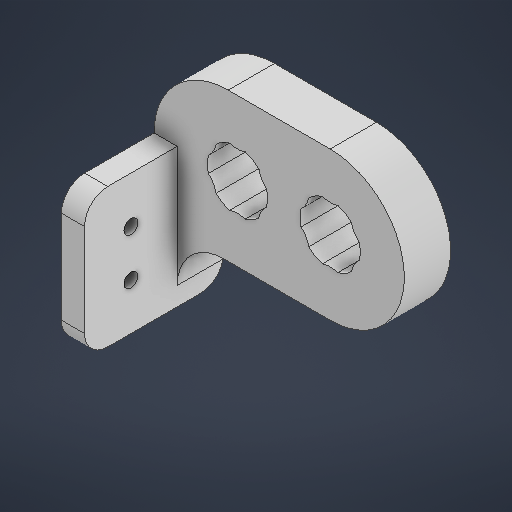
# Autodesk Inventor part: left_holder
Saved by Autodesk Inventor 2026.1 (Build 301233020, 233B)
## iProperties
Created: 2025-12-21
Part Number: left_holder
Material: Ogólny
Document SubType Name: Modeling
Designer: maciej
Density: 1 g/cm^3
Appearance: Domyślna
Author: maciej
Autodesk Inventor part; units mm, degrees
ref_plane "YZ Plane" through (0, 0, 0) normal (1, 0, 0) x (0, 1, 0)
ref_plane "XZ Plane" through (0, 0, 0) normal (0, 1, 0) x (-1, 0, 0)
ref_plane "XY Plane" through (0, 0, 0) normal (0, 0, 1) x (1, 0, 0)
sketch "Sketch1" plane through (0, 0, 0) normal (0, 0, 1) x (1, 0, 0)
  circle A0 centre (0, 0) radius 9.25
  circle A1 centre (0, 30) radius 6
  circle A2 centre (20, 30) radius 6
  circle A3 centre (0, 30) radius 6.5
  circle A4 centre (20, 30) radius 6.5
  arc A5 (-1.6614, 36.2841) -> (1.6614, 36.2841) centre (0, 41) ccw
  arc A6 (-6.2729, 31.7032) -> (-4.6115, 34.5808) centre (-9.5263, 35.5) ccw
  arc A7 (-4.6115, 25.4192) -> (-6.2729, 28.2968) centre (-9.5263, 24.5) ccw
  arc A8 (1.6614, 23.7159) -> (-1.6614, 23.7159) centre (0, 19) ccw
  arc A9 (6.2729, 28.2968) -> (4.6115, 25.4192) centre (9.5263, 24.5) ccw
  arc A10 (4.6115, 34.5808) -> (6.2729, 31.7032) centre (9.5263, 35.5) ccw
  arc A11 (18.3386, 36.2841) -> (21.6614, 36.2841) centre (20, 41) ccw
  arc A12 (13.7271, 31.7032) -> (15.3885, 34.5808) centre (10.4737, 35.5) ccw
  arc A13 (15.3885, 25.4192) -> (13.7271, 28.2968) centre (10.4737, 24.5) ccw
  arc A14 (21.6614, 23.7159) -> (18.3386, 23.7159) centre (20, 19) ccw
  arc A15 (26.2729, 28.2968) -> (24.6115, 25.4192) centre (29.5263, 24.5) ccw
  arc A16 (24.6115, 34.5808) -> (26.2729, 31.7032) centre (29.5263, 35.5) ccw
  arc A17 (4.6562, 34.5353) -> (4.5, 33.9686) centre (20, 30) ccw
  arc A18 (20, 14) -> (20, 46) centre (20, 30) ccw
  line L0 (-18, 30) -> (-18, 0)
  line L1 (-2, 46) -> (20, 46)
  line L2 (-18, 0) -> (-13, 0)
  line L3 (-13, 0) -> (-13, 30)
  line L4 (-13, 30) -> (-18, 30)
  line L5 (-18, 30) -> (-18, 0)
  arc A19 (-2, 46) -> (-18, 30) centre (-2, 30) ccw
  line L6 (20, 14) -> (-13, 14)
  point P0 (15.2791, 25.532)
  point P1 (-18, 30)
  point P2 (-1.6614, 23.7159)
  point P3 (1.6614, 23.7159)
  point P4 (-6.2729, 28.2968)
  point P5 (-4.6115, 25.4192)
  point P6 (-4.6115, 34.5808)
  point P7 (4.635, 34.4629)
  point P8 (6.2729, 31.7032)
  point P9 (18.3386, 23.7159)
  point P10 (21.6614, 23.7159)
  point P11 (13.7271, 31.7032)
  point P12 (26.2729, 31.7032)
  point P13 (15.3885, 25.4192)
  point P14 (15.3885, 34.5808)
  point P15 (4.6115, 25.4192)
  dimension "d1" = 12
  dimension "d0" = 18.5
  dimension "d2" = 30
  dimension "d3" = 12
  dimension "d4" = 20
  dimension "d5" = 13
  dimension "d6" = 13
  dimension "d7" = 5
  dimension "d10" = 360
  dimension "d12" = 5
  dimension "d15" = 360
  dimension "d21" = 16
  dimension "d25" = 5
  dimension "d26" = 30
  dimension "d52" = 18
  constraints: 36 point on circle, 19 centre point, 14 end point, 5 tangent, 4 coincident, 3 horizontal, 3 vertical alignment, 2 horizontal alignment, 2 parallel, 1 perpendicular, 1 point on line, 1 vertical, 54 other
  measures "d0" diameter of A0
  measures "d2" distance of point (0, 0) point (0, 30)
  measures "d3" diameter of A2
  measures "d4" distance of A2.centre point (0, 30)
  measures "d5" diameter of A3
  measures "d6" diameter of A4
  measures "d7" radius of A5
  measures "d12" radius of A11
  measures "d21" radius of A18
  measures "d25" distance of L0.start L3.end
  measures "d26" distance of L3.end L2.end
  measures "d52" distance from line of L0 point (0, 0)
extrude "Extrusion1" add sketch "Sketch1" along normal blind 10 contours A10 A17 A3 | A9 A3 | A8 A3 | A5 A3 | A7 A3 | A6 A3 | A16 A4 | A15 A4 | A11 A4 | A14 A4 | A12 A4 | A13 A4 | L6 L3 L4 A19 L1 A18 | L3 L2 L0 L4 picked at (5.482, 33.1405)
fillet "Fillet2" radius 10 1 edges at (-13, 14, 5)
extrude "Extrusion3" add sketch "Sketch1" along normal blind 30 contours L3 L2 L0 L4
fillet "Fillet3" radius 5 3 edges at (-15.5, 30, 30) (-15.5, 0, 30) (-15.5, 0, 0)
sketch "Sketch3" plane through (-13, 4, 10) normal (1, 0, 0) x (0, 0, -1)
  line L0 (0, 26) -> (-15, 26) projected
  line L1 (-20, 1) -> (-20, 21) projected
  point P0 (10, -4)
  point P1 (-10, 16)
  dimension "d57" = 10
  dimension "d58" = 10
  measures "d57" distance from line of L0 point (-10, 16)
  measures "d58" distance from line of L1 point (-10, 16)
hole "Hole2" at (-13, 20, 20) direction (-1, 0, 0) diameter 3 end through all
sketch "Sketch4" plane through (-13, 4, 10) normal (1, 0, 0) x (0, 0, -1)
  line L0 (5, -4) -> (-15, -4) projected
  line L1 (-20, 1) -> (-20, 21) projected
  point P0 (10, -4)
  point P1 (-10, 6)
  dimension "d66" = 10
  dimension "d67" = 10
  measures "d66" distance from line of L0 point (-10, 6)
  measures "d67" distance from line of L1 point (-10, 6)
hole "Hole3" at (-13, 10, 20) direction (-1, 0, 0) diameter 3 end through all
body "Solid1"
